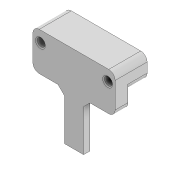
# Autodesk Inventor part: Кронштейн МК
Saved by Autodesk Inventor 2021 (Build 250183000, 183)
## iProperties
Created: 2023-02-18
Part Number: Кронштейн МК
Material: Типовые
Document SubType Name: Modeling
Designer: Tasya
Density: 1 g/cm^3
Appearance: По умолчанию
Mass: 2.38703 g
Surface Area: 16.3431 cm^2
Volume: 2.38703 cm^3
Author: Tasya
Autodesk Inventor part; units mm, degrees
ref_plane "YZ Plane" through (0, 0, 0) normal (1, 0, 0) x (0, 1, 0)
ref_plane "XZ Plane" through (0, 0, 0) normal (0, 1, 0) x (-1, 0, 0)
ref_plane "РабПлоскость1" through (0, -17.25, 7.5) normal (0, 0, 1) x (0, 1, 0)
sketch "Эскиз1" plane through (0, -17.25, 7.5) normal (0, 0, 1) x (0, 1, 0)
  line L0 (17.25, 0) -> (-17.1875, 0) construction
  line L1 (17.25, 10.35) -> (17.25, -10.35) construction
  line L2 (22.25, 12.85) -> (14.25, 12.85)
  line L3 (12.25, 10.85) -> (12.25, -10.85)
  line L4 (14.25, -12.85) -> (22.25, -12.85)
  line L5 (24.25, -10.85) -> (24.25, 10.85)
  line L6 (14.75, -12.85) -> (-9.95, -12.85) construction
  arc A0 (24.25, 10.85) -> (22.25, 12.85) centre (22.25, 10.85) ccw
  arc A1 (22.25, -12.85) -> (24.25, -10.85) centre (22.25, -10.85) ccw
  arc A2 (12.25, -10.85) -> (14.25, -12.85) centre (14.25, -10.85) ccw
  arc A3 (14.25, 12.85) -> (12.25, 10.85) centre (14.25, 10.85) ccw
  point P0 (12.25, -12.85)
  point P1 (12.25, 12.85)
  point P2 (24.25, -12.85)
  dimension "d1" = 5
  dimension "d2" = 12
  dimension "d3" = 2
  dimension "d6" = 2
  constraints: 10 end point, 8 point on circle, 8 tangent, 6 point on line, 4 centre point, 2 equal radius, 2 horizontal, 2 parallel, 1 collinear, 1 perpendicular, 1 other
  measures "d1" distance between parallel lines of L1 L3
  measures "d2" distance of point (12.25, -12.85) point (24.25, -12.85)
  measures "d3" radius of A0
  measures "d6" radius of A2
extrude "Выдавливание1" add sketch "Эскиз1" along normal blind 4
sketch "Эскиз2" plane through (0, -17.25, 7.5) normal (0, 0, -1) x (-1, 0, 0)
  line L0 (10.35, 17.25) -> (-10.35, 17.25) construction
  line L1 (-10.85, 24.25) -> (10.85, 24.25) construction
  line L2 (-12.85, 14.25) -> (-12.85, 22.25) projected
  arc A0 (-12.85, 14.25) -> (-10.85, 12.25) centre (-10.85, 14.25) ccw projected
  line L3 (10.85, 12.25) -> (-10.85, 12.25) construction
  arc A1 (10.85, 12.25) -> (12.85, 14.25) centre (10.85, 14.25) ccw projected
  line L4 (12.85, 22.25) -> (12.85, 14.25) projected
  arc A2 (12.85, 22.25) -> (10.85, 24.25) centre (10.85, 22.25) ccw projected
  line L5 (-10.85, 24.25) -> (10.85, 24.25) projected
  arc A3 (-10.85, 24.25) -> (-12.85, 22.25) centre (-10.85, 22.25) ccw projected
  line L6 (12.85, 17.25) -> (-12.85, 17.25)
  point P0 (0, 17.25)
  point P1 (0, 17.25)
  constraints: 2 end point, 2 midpoint, 2 point on line, 1 horizontal
extrude "Выдавливание2" add sketch "Эскиз2" along normal blind 6
fillet "Сопряжение1" radius 2 2 edges at (-12.85, 0, 4.5) (12.85, 0, 4.5)
sketch "Эскиз3" plane through (0, -17.25, 1.5) normal (0, 0, -1) x (-1, 0, 0)
  arc A0 (-12.85, 19.25) -> (-10.85, 17.25) centre (-10.85, 19.25) ccw construction
  line L0 (-10.85, 17.25) -> (10.85, 17.25) construction
  arc A1 (10.85, 17.25) -> (12.85, 19.25) centre (10.85, 19.25) ccw construction
  line L1 (12.85, 19.25) -> (12.85, 22.25) construction
  arc A2 (12.85, 22.25) -> (10.85, 24.25) centre (10.85, 22.25) ccw construction
  line L2 (10.85, 24.25) -> (-10.85, 24.25) construction
  arc A3 (-10.85, 24.25) -> (-12.85, 22.25) centre (-10.85, 22.25) ccw construction
  line L3 (-12.85, 22.25) -> (-12.85, 19.25) construction
  line L4 (12.85, 20.75) -> (-12.85, 20.75) construction
  line L5 (0, 17.25) -> (0, 28) construction
  point P0 (10.5, 20.75)
  point P1 (-10.5, 20.75)
  dimension "d10" = 21
  constraints: 4 end point, 2 midpoint, 2 point on line, 1 symmetric about line, 1 vertical
  measures "d10" distance of point (10.5, 20.75) point (-10.5, 20.75)
hole "Отверстие1" at (-10.5, 3.5, 1.5) at (10.5, 3.5, 1.5) direction (0, 0, 1) diameter 2.5 depth 4
chamfer "Фаска1" distance 0.2 angle 45 2 edges at (10.5, 2.25, 1.5) (-10.5, 2.25, 1.5)
sketch "Эскиз4" plane through (0, -17.25, 11.5) normal (0, 0, 1) x (1, 0, 0)
  line L0 (0, 17.25) -> (0, -22) construction
  line L1 (-10.85, 12.25) -> (10.85, 12.25) construction
  line L2 (-10.85, 12.25) -> (10.85, 12.25) projected
  line L3 (3, 12.25) -> (-3, 12.25)
  line L4 (-3, 12.25) -> (-3, -2.75)
  line L5 (-3, -2.75) -> (3, -2.75)
  line L6 (3, -2.75) -> (3, 12.25)
  dimension "d21" = 15
  dimension "d22" = 6
  constraints: 10 end point, 2 parallel, 1 horizontal, 1 perpendicular, 1 point on line, 1 vertical, 1 other
  measures "d21" distance of L3.end L4.end
  measures "d22" distance of L4.end L5.end
extrude "Выдавливание3" add sketch "Эскиз4" against normal blind 2
chamfer "Фаска2" distance 2 angle 45 2 edges at (-3, -5, 10.5) (3, -5, 10.5)
sketch "Эскиз5" plane through (0, -17.25, 11.5) normal (0, 0, 1) x (1, 0, 0)
  circle A0 centre (-10.5, 20.75) radius 1.45 projected
  circle A1 centre (10.5, 20.75) radius 1.45 projected
  circle A2 centre (-10.5, 20.75) radius 1.25 projected
  point P0 (0, 17.25)
  constraints: 2 coincident
hole "Отверстие2" at (10.5, 3.5, 11.5) at (-10.5, 3.5, 11.5) direction (0, 0, -1) diameter 2.5 depth 4
chamfer "Фаска3" distance 0.3 angle 45 2 edges at (10.5, 4.75, 11.5) (-10.5, 4.75, 11.5)
